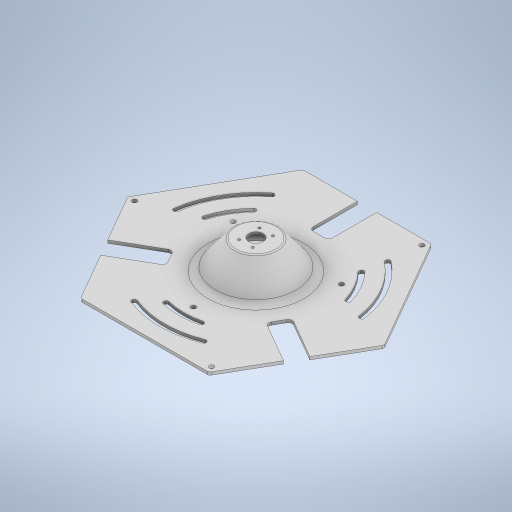
# Autodesk Inventor part: head
Saved by Autodesk Inventor 2023 (Build 270158000, 158)
## iProperties
Created: 2023-11-03
Part Number: head
Material: Ogólny
Document SubType Name: Modeling
Designer: janek
Density: 1 g/cm^3
Appearance: Domyślna
Author: janek
## iProperties of the stored document head_Drukowanie 3D.ipt
Created: 2023-11-13
Part Number: head_Drukowanie 3D
Material: Ogólny
Document SubType Name: Modeling
Designer: janek
Density: 1 g/cm^3
Appearance: Domyślna
Author: janek
Autodesk Inventor part; units mm, degrees
ref_plane "YZ Plane" through (0, 0, 0) normal (1, 0, 0) x (0, 1, 0)
ref_plane "XZ Plane" through (0, 0, 0) normal (0, 1, 0) x (-1, 0, 0)
ref_plane "XY Plane" through (0, 0, 0) normal (0, 0, 1) x (1, 0, 0)
sketch "Szkic1" plane through (0, 0, 0) normal (0, 1, 0) x (-1, 0, 0)
  line L0 (-66.6595, -115.5141) -> (-133.3679, -0.0283)
  line L1 (-133.3679, -0.0283) -> (-66.7084, 115.4859)
  line L2 (-66.7084, 115.4859) -> (66.6595, 115.5141)
  line L3 (66.6595, 115.5141) -> (133.3679, 0.0283)
  line L4 (133.3679, 0.0283) -> (66.7084, -115.4859)
  line L5 (66.7084, -115.4859) -> (-66.6595, -115.5141)
  point P0 (0, 0)
  point P1 (0, 0)
  dimension "d0" = 231
  constraints: 12 end point, 1 coincident, 13 other
  measures "d0" distance between parallel lines of L5 L2
extrude "Wyciągnięcie proste1" add sketch "Szkic1" along normal blind 3
sketch "Szkic2" plane through (0, 3, 0) normal (0, 1, 0) x (1, 0, 0)
  line L0 (-133.3679, -0.0283) -> (-66.6595, -115.5141) projected
  line L1 (-66.7084, 115.4859) -> (-133.3679, -0.0283) projected
  circle A0 centre (63.0524, 109.2634) radius 2.5
  line L2 (66.6595, 115.5141) -> (-66.7084, 115.4859) projected
  line L3 (133.3679, 0.0283) -> (66.6595, 115.5141) projected
  line L4 (66.6595, 115.5141) -> (-66.6595, -115.5141)
  line L5 (-66.6595, -115.5141) -> (66.7084, -115.4859) projected
  line L6 (-66.7084, 115.4859) -> (66.7084, -115.4859)
  line L7 (66.7084, -115.4859) -> (133.3679, 0.0283) projected
  circle A1 centre (63.0987, -109.2366) radius 2.5
  circle A2 centre (-126.151, -0.0267) radius 2.5
  point P0 (0, 0)
  dimension "d10" = 5
  dimension "d13" = 0
  dimension "d14" = 5
  dimension "d18" = 218.5
  dimension "d19" = 5
  dimension "d22" = 218.5
  dimension "d23" = 218.5
  constraints: 4 end point, 3 centre point, 1 point on line
  measures "d10" diameter of A0
  measures "d13" distance from line of L4 A0.centre
  measures "d14" diameter of A1
  measures "d18" distance of A0.centre A1.centre
  measures "d19" diameter of A2
  measures "d22" distance of A2.centre A0.centre
  measures "d23" distance of A2.centre A1.centre
extrude "Wyciągnięcie proste2" cut sketch "Szkic2" against normal blind 3 contours L4 A0 | A0 L4 | A1 L6 | L6 A1 | A2
sketch "Szkic3" plane through (0, 3, 0) normal (0, 1, 0) x (1, 0, 0)
  line L0 (-66.7084, 115.4859) -> (-133.3679, -0.0283) projected
  line L1 (-133.3679, -0.0283) -> (-105.0363, 49.0675)
  line L2 (-133.3679, -0.0283) -> (-66.6595, -115.5141) projected
  line L3 (-105.0155, -49.112) -> (-61.7195, -24.1029)
  line L4 (-61.7195, -24.1029) -> (-51.7159, -41.4213)
  line L5 (-51.7159, -41.4213) -> (-95.0118, -66.4304)
  line L6 (-133.3679, -0.0283) -> (-66.6595, -115.5141) projected
  line L7 (-95.0118, -66.4304) -> (-105.0155, -49.112)
  point P0 (0, 0)
  point P1 (-95.0118, -66.4304)
  dimension "d24" = 56.684
  dimension "d25" = 50
  dimension "d26" = 20
  dimension "d54" = 56.684
  dimension "d55" = 56.6839
  constraints: 10 end point, 3 perpendicular, 2 point on line, 1 collinear
  measures "d24" distance of L0.end L1.end
  measures "d25" distance of L3.start L3.end
  measures "d26" distance of L3.end L4.end
  measures "d54" distance of L0.end L3.start
  measures "d55" distance of L5.end L2.end
extrude "Wyciągnięcie proste3" cut sketch "Szkic3" against normal blind 3
sketch "Szkic4" plane through (0, 3, 0) normal (0, 1, 0) x (1, 0, 0)
  line L0 (66.7084, -115.4859) -> (133.3679, 0.0283) projected
  line L1 (66.7084, -115.4859) -> (95.04, -66.3901)
  line L2 (95.04, -66.3901) -> (51.7335, -41.3992)
  line L3 (51.7335, -41.3992) -> (61.7298, -24.0766)
  line L4 (61.7298, -24.0766) -> (105.0364, -49.0674)
  line L5 (105.0364, -49.0674) -> (95.04, -66.3901)
  point P0 (0, 0)
  dimension "d29" = 56.684
  dimension "d30" = 50
  dimension "d31" = 20
  constraints: 10 end point, 4 perpendicular, 2 point on line
  measures "d29" distance of L0.start L1.end
  measures "d30" distance of L1.end L2.end
  measures "d31" distance of L2.end L3.end
extrude "Wyciągnięcie proste4" cut sketch "Szkic4" against normal blind 3
sketch "Szkic5" plane through (0, 3, 0) normal (0, 1, 0) x (1, 0, 0)
  line L0 (66.6595, 115.5141) -> (9.9755, 115.5021)
  line L1 (66.6595, 115.5141) -> (-66.7084, 115.4859) projected
  line L2 (9.9755, 115.5021) -> (9.9861, 65.5021)
  line L3 (9.9861, 65.5021) -> (-10.0139, 65.4979)
  line L4 (-10.0139, 65.4979) -> (-10.0245, 115.4979)
  line L5 (9.9755, 115.5021) -> (-10.0245, 115.4979)
  point P0 (0, 0)
  dimension "d34" = 56.684
  dimension "d35" = 50
  dimension "d36" = 20
  constraints: 10 end point, 4 perpendicular, 2 point on line
  measures "d34" distance of L0.start L0.end
  measures "d35" distance of L0.end L2.end
  measures "d36" distance of L2.end L3.end
extrude "Wyciągnięcie proste5" cut sketch "Szkic5" against normal blind 3
sketch "Szkic6" plane through (0, 3, 0) normal (0, 1, 0) x (1, 0, 0)
  circle A0 centre (0, 0) radius 100
  circle A1 centre (0, 0) radius 95
  line L0 (-95.0118, -66.4304) -> (-51.7159, -41.4213) projected
  line L1 (-76.8035, -55.9127) -> (76.8272, -55.88)
  line L2 (51.7335, -41.3992) -> (95.04, -66.3901) projected
  line L3 (-105.0155, -49.112) -> (-61.7195, -24.1029) projected
  line L4 (-86.8071, -38.5943) -> (-10.0201, 94.4701)
  line L5 (-10.0245, 115.4979) -> (-10.0139, 65.4979) projected
  line L6 (9.9861, 65.5021) -> (9.9755, 115.5021) projected
  line L7 (9.9799, 94.4743) -> (86.8235, -38.5574)
  line L8 (105.0364, -49.0674) -> (61.7298, -24.0766) projected
  line L9 (-91.1597, -41.1085) -> (-86.8071, -38.5943)
  line L10 (-81.156, -58.4269) -> (-76.8035, -55.9127)
  line L11 (76.8272, -55.88) -> (81.1808, -58.3924)
  line L12 (86.8235, -38.5574) -> (91.1772, -41.0697)
  line L13 (9.9789, 99.5009) -> (9.9799, 94.4743)
  line L14 (-10.0211, 99.4966) -> (-10.0201, 94.4701)
  line L15 (48.4019, 27.9582) -> (94.3313, 11.252)
  line L16 (48.4019, 27.9582) -> (56.8787, 76.0908)
  line L17 (56.8787, 76.0908) -> (59.3946, 80.4505)
  line L18 (94.3313, 11.252) -> (99.3649, 11.252)
  circle A2 centre (0, 0) radius 80
  circle A3 centre (0, 0) radius 75
  line L19 (72.5029, 19.1917) -> (77.6639, 19.1917)
  line L20 (52.85, 53.2153) -> (55.4294, 57.6852)
  line L21 (-48.4163, 27.9333) -> (-56.9179, 76.0615)
  line L22 (-48.4163, 27.9333) -> (-94.3371, 11.2034)
  line L23 (-56.9179, 76.0615) -> (-60.0082, 79.9938)
  line L24 (-94.3371, 11.2034) -> (-99.3704, 11.2034)
  line L25 (-72.5128, 19.1544) -> (-77.559, 19.6112)
  line L26 (-52.8774, 53.1881) -> (-55.9867, 57.1445)
  line L27 (0.0119, -55.8964) -> (-37.4206, -87.3195)
  line L28 (0.0119, -55.8964) -> (37.4577, -87.3036)
  line L29 (-19.6305, -72.3854) -> (-21.3764, -77.0912)
  line L30 (19.6613, -72.377) -> (21.3764, -77.0912)
  line L31 (-37.4206, -87.3195) -> (-39.1619, -92.0128)
  line L32 (37.4577, -87.3036) -> (39.1698, -92.0094)
  dimension "d39" = 200
  dimension "d40" = 190
  dimension "d42" = 76.815
  dimension "d43" = 100
  dimension "d44" = 160
  dimension "d45" = 150
  dimension "d46" = 76.81
  dimension "d47" = 100
  dimension "d48" = 100
  constraints: 54 end point, 20 point on line, 12 point on circle, 4 coincident, 4 parallel, 3 collinear, 3 equal length, 3 horizontal, 2 centre point, 1 midpoint, 28 other
  measures "d42" distance of L15.start L7.end
  measures "d43" angle of L15 L16
  measures "d44" diameter of A2
  measures "d45" diameter of A3
  measures "d46" distance of L4.start L21.start
  measures "d47" angle of L21 L22
  measures "d48" angle of L28 L27
extrude "Wyciągnięcie proste6" cut sketch "Szkic6" against normal blind 10 contours L18 A1 L17 A0 | A0 L31 A1 L32 | A3 L20 A2 L19 | L23 A1 L24 A0 | A2 L29 A3 L30 | L26 A3 L25 A2
sketch "Szkic7" plane through (0, 3, 0) normal (0, 1, 0) x (1, 0, 0)
  point P0 (0, 0)
fillet "Zaokrąglenie1" radius 3 6 edges at (66.6595, 1.5, -115.5141) (133.3679, 1.5, -0.0283) (66.7084, 1.5, 115.4859) (-66.6595, 1.5, 115.5141) (-133.3679, 1.5, 0.0283) (-66.7084, 1.5, -115.4859)
fillet "Zaokrąglenie2" radius 4 6 edges at (-10.0139, 1.5, -65.4979) (9.9861, 1.5, -65.5021) (-51.7159, 1.5, 41.4213) (-61.7195, 1.5, 24.1029) (51.7335, 1.5, 41.3992) (61.7298, 1.5, 24.0766)
fillet "Zaokrąglenie3" radius 2 24 edges at (-99.3704, 1.5, -11.2034) (-94.3371, 1.5, -11.2034) (-72.5128, 1.5, -19.1544) (21.3764, 1.5, 77.0912) (39.1698, 1.5, 92.0094) (19.6613, 1.5, 72.377) (37.4577, 1.5, 87.3036) (-55.9867, 1.5, -57.1445) (-60.0082, 1.5, -79.9938) (-52.8774, 1.5, -53.1881) (-56.9179, 1.5, -76.0615) (-77.559, 1.5, -19.6112) (52.85, 1.5, -53.2153) (56.8787, 1.5, -76.0908) (72.5029, 1.5, -19.1917) (94.3313, 1.5, -11.252) (-39.1619, 1.5, 92.0128) (-21.3764, 1.5, 77.0912) (-19.6305, 1.5, 72.3854) (-37.4206, 1.5, 87.3195) (55.4294, 1.5, -57.6852) (59.3946, 1.5, -80.4505) (77.6639, 1.5, -19.1917) (99.3649, 1.5, -11.252)
sketch "Szkic9" plane through (0, 3, 0) normal (0, 1, 0) x (1, 0, 0)
  circle A0 centre (0, 0) radius 45
  dimension "d57" = 90
  constraints: 1 centre point, 1 coincident
  measures "d57" diameter of A0
extrude "Wyciągnięcie proste7" add sketch "Szkic9" along normal blind 30
sketch "Szkic10" plane through (0, 33, 0) normal (0, 1, 0) x (1, 0, 0)
  line L0 (-7, 10.5) -> (7, 10.5)
  line L1 (7, 10.5) -> (7, -10.5)
  line L2 (7, -10.5) -> (-7, -10.5)
  line L3 (-7, -10.5) -> (-7, 10.5)
  line L4 (-7, 10.5) -> (7, -10.5) construction
  line L5 (7, 10.5) -> (-7, -10.5) construction
  circle A0 centre (-7, 10.5) radius 1.25
  circle A1 centre (7, 10.5) radius 1.25
  circle A2 centre (-7, -10.5) radius 1.25
  circle A3 centre (7, -10.5) radius 1.25
  circle A4 centre (0, 0) radius 7.5
  point P0 (0, 10.5)
  point P1 (0, -10.5)
  dimension "d60" = 14
  dimension "d61" = 21
  dimension "d62" = 2.5
  dimension "d63" = 2.5
  dimension "d64" = 2.5
  dimension "d65" = 2.5
  dimension "d76" = 15
  constraints: 12 end point, 5 centre point, 5 coincident, 4 midpoint, 2 parallel, 1 horizontal, 1 perpendicular
  measures "d60" distance of L1.end L2.end
  measures "d61" distance of point (0, 10.5) point (0, -10.5)
  measures "d62" diameter of A0
  measures "d63" diameter of A1
  measures "d64" diameter of A2
  measures "d65" diameter of A3
  measures "d76" diameter of A4
chamfer "Faza1" distance 30 angle 38 1 edges at (-45, 33, 0) measured on face at (-45, 32.5, 0)
sketch "Szkic11" plane through (0, 0, 0) normal (0, -1, 0) x (1, 0, 0)
  circle A0 centre (0, 0) radius 17.5
  dimension "d69" = 35
  constraints: 1 centre point, 1 coincident
  measures "d69" diameter of A0
extrude "Wyciągnięcie proste8" cut sketch "Szkic11" against normal blind 30
chamfer "Faza2" distance 23 distance2 30 1 edges at (-17.5, 0, 0) measured on face at (-18, 0, 0)
fillet "Zaokrąglenie4" radius 10 1 edges at (-40.4999, 0, 0)
extrude "Wyciągnięcie proste9" cut sketch "Szkic10" against normal blind 30 contours A4 L1 L3 | L3 A4 | A4 L1
extrude "Wyciągnięcie proste10" cut sketch "Szkic10" against normal blind 30 contours L3 A0 L0 | L0 A0 L3 | A1 L1 L0 | L0 L1 A1 | A2 L2 L3 | L3 L2 A2 | A3 L2 L1 | L1 L2 A3
fillet "Zaokrąglenie5" radius 10 2 edges at (-45, 3, 0) (-45, 3.0001, 0)
sketch "Szkic12" plane through (0, 0, 0) normal (0, -1, 0) x (1, 0, 0)
  circle A0 centre (56.2874, -32.5073) radius 2.5
  circle A1 centre (0.0082, 65) radius 2.5
  circle A2 centre (-56.2959, -32.4929) radius 2.5
  line L0 (0.0082, 65) -> (56.2874, -32.5073)
  line L1 (-56.2959, -32.4929) -> (56.2874, -32.5073)
  line L2 (-56.2959, -32.4929) -> (0.0082, 65)
  arc A3 (17.9251, 72.8264) -> (-17.9058, 72.8312) centre (0, 0) ccw projected
  arc A4 (53.9064, -52.145) -> (72.1037, -20.6413) centre (0, 0) ccw projected
  arc A5 (-72.0742, -20.7437) -> (-54.0943, -51.95) centre (0, 0) ccw projected
  line L3 (0.0099, 75) -> (-0.0139, -65.5)
  line L4 (5.9861, -65.5013) -> (-6.0139, -65.4987) projected
  point P0 (64.9442, -37.5133)
  point P1 (-64.9853, -37.4422)
  dimension "d82" = 60
  dimension "d83" = 60
  dimension "d84" = 10
  dimension "d85" = 10
  dimension "d86" = 10
  dimension "d87" = 5
  dimension "d88" = 5
  dimension "d89" = 5
  constraints: 8 end point, 3 centre point, 3 point on circle, 1 midpoint, 1 point on line
  measures "d82" angle of L0 L2
  measures "d83" angle of L1 L0
  measures "d84" distance of L3.start L0.start
  measures "d85" distance of point (64.944, -37.513) L0.end
  measures "d86" distance of point (-64.985, -37.442) L1.start
  measures "d87" diameter of A1
  measures "d88" diameter of A0
  measures "d89" diameter of A2
extrude "Wyciągnięcie proste11" cut sketch "Szkic12" against normal blind 10 contours A0 L1 L0 | L0 L1 A0 | L0 L3 A1 | A1 L3 L0 | A1 L2 L3 | L2 A1 L3 | L1 L2 A2 | A2 L2 L1
fillet "Zaokrąglenie6" radius 2 2 edges at (-17.5, 29.9999, 0) (-17.5, 30, 0)
fillet "Zaokrąglenie7" radius 2 1 edges at (-21.5615, 33, 0)
